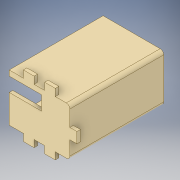
# Autodesk Inventor part: Case_Body
Saved by Autodesk Inventor 2019 (Build 230136000, 136)
## iProperties
Created: 2019-02-19
Part Number: Case_Body
Material: 일반
Document SubType Name: Modeling
Designer: Jeong Ji Hoon
Density: 1 g/cm^3
Appearance: 베이지색
Author: Jeong Ji Hoon
## iProperties of the stored document Case_Body_3D 인쇄.ipt
Created: 2019-02-22
Part Number: Case_Body_3D 인쇄
Material: 일반
Document SubType Name: Modeling
Designer: Jeong Ji Hoon
Density: 1 g/cm^3
Appearance: 기본값
Author: Jeong Ji Hoon
Autodesk Inventor part; units mm, degrees
ref_plane "YZ Plane" through (0, 0, 0) normal (1, 0, 0) x (0, 1, 0)
ref_plane "XZ Plane" through (0, 0, 0) normal (0, 1, 0) x (-1, 0, 0)
ref_plane "XY Plane" through (0, 0, 0) normal (0, 0, 1) x (1, 0, 0)
sketch "스케치1" plane through (0, 0, 0) normal (0, 0, 1) x (1, 0, 0)
  line L0 (0, 0) -> (18.6, 0)
  line L1 (18.6, 0) -> (18.6, 13.5)
  line L2 (18.6, 13.5) -> (0, 13.5)
  line L3 (0, 13.5) -> (0, 0)
  line L4 (1.5, 12) -> (17.1, 12)
  line L5 (17.1, 12) -> (17.1, 1.5)
  line L6 (17.1, 1.5) -> (1.5, 1.5)
  line L7 (1.5, 1.5) -> (1.5, 12)
  dimension "d4" = 18.6
  dimension "d5" = 13.5
  dimension "d6" = 1.5
  constraints: 16 end point, 4 parallel, 2 perpendicular, 1 horizontal, 3 other
  measures "d4" distance of L2.end L1.end
  measures "d5" distance of L0.end L1.end
  measures "d6" distance between parallel lines of L2 L4
extrude "돌출1" add sketch "스케치1" along normal blind 25.5
sketch "스케치2" plane through (0, 0, 25.5) normal (0, 0, 1) x (1, 0, 0)
  line L0 (0, 0) -> (18.6, 0) projected
  line L1 (18.6, 0) -> (18.6, 13.5) projected
  line L2 (0, 0) -> (18.6, 0)
  line L3 (18.6, 0) -> (18.6, 8)
  line L4 (18.6, 8) -> (0, 8)
  line L5 (0, 8) -> (0, 0)
  line L6 (18.6, 13.5) -> (0, 13.5) projected
  line L7 (18.6, 8) -> (10.6, 8)
  line L8 (10.6, 8) -> (10.6, 13.5)
  line L9 (10.6, 13.5) -> (18.6, 13.5)
  line L10 (18.6, 13.5) -> (18.6, 8)
  line L11 (0, 13.5) -> (0, 0) projected
  line L12 (17.1, 12) -> (1.5, 12) projected
  line L13 (0, 13.5) -> (10.6, 13.5)
  line L14 (10.6, 13.5) -> (10.6, 12)
  line L15 (10.6, 12) -> (0, 12)
  line L16 (0, 12) -> (0, 13.5)
  dimension "d9" = 8
  dimension "d14" = 8
  constraints: 24 end point, 6 parallel, 4 point on line, 3 horizontal, 3 perpendicular
  measures "d9" distance between parallel lines of L0 L4
  measures "d14" distance between parallel lines of L1 L8
extrude "돌출2" add sketch "스케치2" along normal blind 1 contours L5 L4 L1 L0 | L4 L8 L6 L1 | L11 L6 L8 L12 L15
sketch "스케치3" plane through (0, 0, 0) normal (0, 0, -1) x (-1, 0, 0)
  line L0 (-17.1, 1.5) -> (-17.1, 12) projected
  line L1 (-17.1, 12) -> (-1.5, 12) projected
  line L2 (-1.5, 12) -> (-1.5, 1.5) projected
  line L3 (-1.5, 1.5) -> (-17.1, 1.5) projected
  line L4 (0, 0) -> (-18.6, 0) projected
  line L5 (0, 13.5) -> (0, 0) projected
  line L6 (-18.6, 13.5) -> (0, 13.5) projected
  line L7 (-18.6, 0) -> (-18.6, 13.5) projected
  line L8 (-18.6, 13.5) -> (0, 13.5) projected
  line L9 (0, 0) -> (-1.5, 0)
  line L10 (-1.5, 0) -> (-1.5, 13.5)
  line L11 (-1.5, 13.5) -> (0, 13.5)
  line L12 (0, 13.5) -> (0, 0)
  point P0 (-1.5, 6.75)
  constraints: 8 end point, 2 parallel, 1 horizontal, 1 midpoint, 1 perpendicular, 1 point on line, 1 vertical alignment
extrude "돌출3" cut sketch "스케치3" against normal up to next contours L2 L10 L6 L5 L4
sketch "스케치4" plane through (18.6, 0, 0) normal (0, -1, 0) x (1, 0, 0)
  line L0 (-7.8, 21) -> (-17.1, 21)
  line L1 (-17.1, 21) -> (-17.1, 21.5)
  line L2 (-17.1, 21.5) -> (-7.8, 21.5)
  line L3 (-7.8, 21.5) -> (-7.8, 21)
  line L4 (-17.1, 26.5) -> (-17.1, 0) projected
  line L5 (-17.1, 26.5) -> (0, 26.5) projected
  point P0 (-18.6, 0)
  dimension "d17" = 0.5
  dimension "d18" = 9.3
  dimension "d19" = 5
  constraints: 8 end point, 2 parallel, 1 collinear, 1 horizontal, 1 perpendicular
  measures "d17" distance of L0.end L1.end
  measures "d18" distance of L0.start L0.end
  measures "d19" distance between parallel lines of L2 L5
extrude "돌출4" cut sketch "스케치4" against normal up to next
sketch "스케치5" plane through (18.6, 13.5, 26.5) normal (0, 1, 0) x (1, 0, 0)
  line L0 (-13.1, 0) -> (-10.1, 0)
  line L1 (-10.1, 0) -> (-10.1, 1)
  line L2 (-10.1, 1) -> (-13.1, 1)
  line L3 (-13.1, 1) -> (-13.1, 0)
  line L4 (-17.1, 26.5) -> (-17.1, 0) projected
  line L5 (0, 0) -> (-17.1, 0) projected
  line L6 (-7.1, 0) -> (-4.1, 0)
  line L7 (-4.1, 0) -> (-4.1, 1)
  line L8 (-4.1, 1) -> (-7.1, 1)
  line L9 (-7.1, 1) -> (-7.1, 0)
  point P0 (-18.6, 26.5)
  dimension "d20" = 1
  dimension "d21" = 3
  dimension "d22" = 4
  dimension "d23" = 3
  dimension "d24" = 1
  dimension "d25" = 3
  constraints: 16 end point, 4 parallel, 2 horizontal, 2 perpendicular, 1 collinear, 1 point on line
  measures "d20" distance of L0.end L1.end
  measures "d21" distance of L1.end L2.end
  measures "d22" distance between parallel lines of L4 L3
  measures "d23" distance of L8.end L7.end
  measures "d24" distance of L7.end L6.end
  measures "d25" distance between parallel lines of L1 L9
extrude "돌출5" add sketch "스케치5" along normal blind 2
sketch "스케치6" plane through (18.6, 0, 0) normal (1, 0, 0) x (0, 0, -1)
  line L0 (-26.5, 0) -> (-26.5, 13.5) projected
  line L1 (-26.5, 5) -> (-25.5, 5)
  line L2 (-25.5, 5) -> (-25.5, 8)
  line L3 (-25.5, 8) -> (-26.5, 8)
  line L4 (-26.5, 8) -> (-26.5, 5)
  line L5 (0, 0) -> (-26.5, 0) projected
  dimension "d28" = 1
  dimension "d29" = 3
  dimension "d30" = 5
  constraints: 8 end point, 2 parallel, 1 horizontal, 1 perpendicular, 1 point on line
  measures "d28" distance of L3.end L2.end
  measures "d29" distance of L2.end L1.end
  measures "d30" distance between parallel lines of L5 L1
extrude "돌출6" add sketch "스케치6" along normal blind 2
fillet "모깎기1" radius 1 2 edges at (18.6, 13.5, 13.25) (18.6, 0, 13.25)
sketch "스케치11" plane through (1.5, 12, 0) normal (-1, 0, 0) x (0, 0, 1)
  line L0 (1, 0.75) -> (2, 0.75)
  line L1 (2, 0.75) -> (2, -11.25)
  line L2 (2, -11.25) -> (1, -11.25)
  line L3 (1, -11.25) -> (1, 0.75)
  line L4 (0, -10.5) -> (0, 0) projected
  line L5 (0, 1.5) -> (26.5, 1.5) projected
  line L6 (21, -12) -> (0, -12) projected
  dimension "d43" = 1
  dimension "d44" = 1
  dimension "d45" = 0.75
  dimension "d46" = 0.75
  constraints: 8 end point, 2 parallel, 1 horizontal, 1 perpendicular
  measures "d43" distance of L1.end L2.end
  measures "d44" distance between parallel lines of L4 L3
  measures "d45" distance between parallel lines of L5 L0
  measures "d46" distance between parallel lines of L2 L6
extrude "돌출8" cut sketch "스케치11" against normal blind 16.1
sketch "스케치12" plane through (1.5, 0, 21.5) normal (0, -1, 0) x (1, 0, 0)
  line L0 (13, 4) -> (10, 4)
  line L1 (10, 4) -> (10, 5)
  line L2 (10, 5) -> (13, 5)
  line L3 (13, 5) -> (13, 4)
  line L4 (0, 5) -> (16.1, 5) projected
  line L5 (17.1, -21.5) -> (17.1, 5) projected
  line L6 (9.1, 5) -> (0, 5) projected
  line L7 (7, 5) -> (4, 5)
  line L8 (4, 5) -> (4, 4)
  line L9 (4, 4) -> (7, 4)
  line L10 (7, 4) -> (7, 5)
  line L11 (0, 5) -> (0, 0) projected
  point P0 (-1.5, -21.5)
  dimension "d49" = 3
  dimension "d50" = 1
  dimension "d52" = 3
  dimension "d53" = 1
  dimension "d54" = 3
  dimension "d55" = 4
  constraints: 16 end point, 4 parallel, 2 horizontal, 2 perpendicular, 1 collinear, 1 point on line
  measures "d49" distance of L1.end L2.end
  measures "d50" distance of L0.end L1.end
  measures "d52" distance of L9.end L8.end
  measures "d53" distance of L8.end L7.end
  measures "d54" distance between parallel lines of L1 L10
  measures "d55" distance between parallel lines of L8 L11
extrude "돌출9" add sketch "스케치12" along normal blind 2
equation "\"d6\" = t"
equation "\"t\" = 1.5"
